Autodesk Fusion 360 part; units mm, degrees
(part 5 of 12)
sketch "草图29" plane through (-71.4999, -0.0001, 0) normal (-1, -0.000001, 0) x (0.000001, -1, 0)
  line L0 (-161.5001, 0) -> (74.9986, 0)
  line L1 (74.9986, 0) -> (74.9986, 250)
  line L2 (74.9986, 250) -> (-161.5001, 250)
  line L3 (-161.5001, 250) -> (-161.5001, 0)
  line L4 (-151.5001, 15) -> (-155.8302, 12.5)
  line L5 (-155.8302, 12.5) -> (-155.8302, 7.5)
  line L6 (-155.8302, 7.5) -> (-151.5001, 5)
  line L7 (-151.5001, 5) -> (-147.17, 7.5)
  line L8 (-147.17, 7.5) -> (-147.17, 12.5)
  line L9 (-147.17, 12.5) -> (-151.5001, 15)
  line L10 (-140.8398, 15) -> (-145.17, 12.5)
  line L11 (-145.17, 12.5) -> (-145.17, 7.5)
  line L12 (-145.17, 7.5) -> (-140.8398, 5)
  line L13 (-140.8398, 5) -> (-136.5097, 7.5)
  line L14 (-136.5097, 7.5) -> (-136.5097, 12.5)
  line L15 (-136.5097, 12.5) -> (-140.8398, 15)
  line L16 (-130.1796, 15) -> (-134.5097, 12.5)
  line L17 (-134.5097, 12.5) -> (-134.5097, 7.5)
  line L18 (-134.5097, 7.5) -> (-130.1796, 5)
  line L19 (-130.1796, 5) -> (-125.8494, 7.5)
  line L20 (-125.8494, 7.5) -> (-125.8494, 12.5)
  line L21 (-125.8494, 12.5) -> (-130.1796, 15)
  line L22 (-119.5193, 15) -> (-123.8494, 12.5)
  line L23 (-123.8494, 12.5) -> (-123.8494, 7.5)
  line L24 (-123.8494, 7.5) -> (-119.5193, 5)
  line L25 (-119.5193, 5) -> (-115.1892, 7.5)
  line L26 (-115.1892, 7.5) -> (-115.1892, 12.5)
  line L27 (-115.1892, 12.5) -> (-119.5193, 15)
  line L28 (-108.8591, 15) -> (-113.1892, 12.5)
  line L29 (-113.1892, 12.5) -> (-113.1892, 7.5)
  line L30 (-113.1892, 7.5) -> (-108.8591, 5)
  line L31 (-108.8591, 5) -> (-104.5289, 7.5)
  line L32 (-104.5289, 7.5) -> (-104.5289, 12.5)
  line L33 (-104.5289, 12.5) -> (-108.8591, 15)
  line L34 (-98.1988, 15) -> (-102.5289, 12.5)
  line L35 (-102.5289, 12.5) -> (-102.5289, 7.5)
  line L36 (-102.5289, 7.5) -> (-98.1988, 5)
  line L37 (-98.1988, 5) -> (-93.8687, 7.5)
  line L38 (-93.8687, 7.5) -> (-93.8687, 12.5)
  line L39 (-93.8687, 12.5) -> (-98.1988, 15)
  line L40 (-87.5386, 15) -> (-91.8687, 12.5)
  line L41 (-91.8687, 12.5) -> (-91.8687, 7.5)
  line L42 (-91.8687, 7.5) -> (-87.5386, 5)
  line L43 (-87.5386, 5) -> (-83.2084, 7.5)
  line L44 (-83.2084, 7.5) -> (-83.2084, 12.5)
  line L45 (-83.2084, 12.5) -> (-87.5386, 15)
  line L46 (-76.8783, 15) -> (-81.2084, 12.5)
  line L47 (-81.2084, 12.5) -> (-81.2084, 7.5)
  line L48 (-81.2084, 7.5) -> (-76.8783, 5)
  line L49 (-76.8783, 5) -> (-72.5482, 7.5)
  line L50 (-72.5482, 7.5) -> (-72.5482, 12.5)
  line L51 (-72.5482, 12.5) -> (-76.8783, 15)
  line L52 (-66.218, 15) -> (-70.5482, 12.5)
  line L53 (-70.5482, 12.5) -> (-70.5482, 7.5)
  line L54 (-70.5482, 7.5) -> (-66.218, 5)
  line L55 (-66.218, 5) -> (-61.8879, 7.5)
  line L56 (-61.8879, 7.5) -> (-61.8879, 12.5)
  line L57 (-61.8879, 12.5) -> (-66.218, 15)
  line L58 (-55.5578, 15) -> (-59.8879, 12.5)
  line L59 (-59.8879, 12.5) -> (-59.8879, 7.5)
  line L60 (-59.8879, 7.5) -> (-55.5578, 5)
  line L61 (-55.5578, 5) -> (-51.2277, 7.5)
  line L62 (-51.2277, 7.5) -> (-51.2277, 12.5)
  line L63 (-51.2277, 12.5) -> (-55.5578, 15)
  line L64 (-44.8975, 15) -> (-49.2277, 12.5)
  line L65 (-49.2277, 12.5) -> (-49.2277, 7.5)
  line L66 (-49.2277, 7.5) -> (-44.8975, 5)
  line L67 (-44.8975, 5) -> (-40.5674, 7.5)
  line L68 (-40.5674, 7.5) -> (-40.5674, 12.5)
  line L69 (-40.5674, 12.5) -> (-44.8975, 15)
  line L70 (-34.2373, 15) -> (-38.5674, 12.5)
  line L71 (-38.5674, 12.5) -> (-38.5674, 7.5)
  line L72 (-38.5674, 7.5) -> (-34.2373, 5)
  line L73 (-34.2373, 5) -> (-29.9072, 7.5)
  line L74 (-29.9072, 7.5) -> (-29.9072, 12.5)
  line L75 (-29.9072, 12.5) -> (-34.2373, 15)
  line L76 (-23.577, 15) -> (-27.9072, 12.5)
  line L77 (-27.9072, 12.5) -> (-27.9072, 7.5)
  line L78 (-27.9072, 7.5) -> (-23.577, 5)
  line L79 (-23.577, 5) -> (-19.2469, 7.5)
  line L80 (-19.2469, 7.5) -> (-19.2469, 12.5)
  line L81 (-19.2469, 12.5) -> (-23.577, 15)
  line L82 (-12.9168, 15) -> (-17.2469, 12.5)
  line L83 (-17.2469, 12.5) -> (-17.2469, 7.5)
  line L84 (-17.2469, 7.5) -> (-12.9168, 5)
  line L85 (-12.9168, 5) -> (-8.5866, 7.5)
  line L86 (-8.5866, 7.5) -> (-8.5866, 12.5)
  line L87 (-8.5866, 12.5) -> (-12.9168, 15)
  line L88 (-2.2565, 15) -> (-6.5866, 12.5)
  line L89 (-6.5866, 12.5) -> (-6.5866, 7.5)
  line L90 (-6.5866, 7.5) -> (-2.2565, 5)
  line L91 (-2.2565, 5) -> (2.0736, 7.5)
  line L92 (2.0736, 7.5) -> (2.0736, 12.5)
  line L93 (2.0736, 12.5) -> (-2.2565, 15)
  line L94 (8.4037, 15) -> (4.0736, 12.5)
  line L95 (4.0736, 12.5) -> (4.0736, 7.5)
  line L96 (4.0736, 7.5) -> (8.4037, 5)
  line L97 (8.4037, 5) -> (12.7339, 7.5)
  line L98 (12.7339, 7.5) -> (12.7339, 12.5)
  line L99 (12.7339, 12.5) -> (8.4037, 15)
  line L100 (19.064, 15) -> (14.7339, 12.5)
  line L101 (14.7339, 12.5) -> (14.7339, 7.5)
  line L102 (14.7339, 7.5) -> (19.064, 5)
  line L103 (19.064, 5) -> (23.3941, 7.5)
  line L104 (23.3941, 7.5) -> (23.3941, 12.5)
  line L105 (23.3941, 12.5) -> (19.064, 15)
  line L106 (29.7242, 15) -> (25.3941, 12.5)
  line L107 (25.3941, 12.5) -> (25.3941, 7.5)
  line L108 (25.3941, 7.5) -> (29.7242, 5)
  line L109 (29.7242, 5) -> (34.0544, 7.5)
  line L110 (34.0544, 7.5) -> (34.0544, 12.5)
  line L111 (34.0544, 12.5) -> (29.7242, 15)
  line L112 (40.3845, 15) -> (36.0544, 12.5)
  line L113 (36.0544, 12.5) -> (36.0544, 7.5)
  line L114 (36.0544, 7.5) -> (40.3845, 5)
  line L115 (40.3845, 5) -> (44.7146, 7.5)
  line L116 (44.7146, 7.5) -> (44.7146, 12.5)
  line L117 (44.7146, 12.5) -> (40.3845, 15)
  line L118 (51.0447, 15) -> (46.7146, 12.5)
  line L119 (46.7146, 12.5) -> (46.7146, 7.5)
  line L120 (46.7146, 7.5) -> (51.0447, 5)
  line L121 (51.0447, 5) -> (55.3749, 7.5)
  line L122 (55.3749, 7.5) -> (55.3749, 12.5)
  line L123 (55.3749, 12.5) -> (51.0447, 15)
  line L124 (61.705, 15) -> (57.3749, 12.5)
  line L125 (57.3749, 12.5) -> (57.3749, 7.5)
  line L126 (57.3749, 7.5) -> (61.705, 5)
  line L127 (61.705, 5) -> (66.0351, 7.5)
  line L128 (66.0351, 7.5) -> (66.0351, 12.5)
  line L129 (66.0351, 12.5) -> (61.705, 15)
  line L130 (-146.17, 24.2321) -> (-150.5001, 21.7321)
  line L131 (-150.5001, 21.7321) -> (-150.5001, 16.7321)
  line L132 (-150.5001, 16.7321) -> (-146.17, 14.2321)
  line L133 (-146.17, 14.2321) -> (-141.8398, 16.7321)
  line L134 (-141.8398, 16.7321) -> (-141.8398, 21.7321)
  line L135 (-141.8398, 21.7321) -> (-146.17, 24.2321)
  line L136 (-135.5097, 24.2321) -> (-139.8398, 21.7321)
  line L137 (-139.8398, 21.7321) -> (-139.8398, 16.7321)
  line L138 (-139.8398, 16.7321) -> (-135.5097, 14.2321)
  line L139 (-135.5097, 14.2321) -> (-131.1796, 16.7321)
  line L140 (-131.1796, 16.7321) -> (-131.1796, 21.7321)
  line L141 (-131.1796, 21.7321) -> (-135.5097, 24.2321)
  line L142 (-124.8494, 24.2321) -> (-129.1796, 21.7321)
  line L143 (-129.1796, 21.7321) -> (-129.1796, 16.7321)
  line L144 (-129.1796, 16.7321) -> (-124.8494, 14.2321)
  line L145 (-124.8494, 14.2321) -> (-120.5193, 16.7321)
  line L146 (-120.5193, 16.7321) -> (-120.5193, 21.7321)
  line L147 (-120.5193, 21.7321) -> (-124.8494, 24.2321)
  line L148 (-114.1892, 24.2321) -> (-118.5193, 21.7321)
  line L149 (-118.5193, 21.7321) -> (-118.5193, 16.7321)
  line L150 (-118.5193, 16.7321) -> (-114.1892, 14.2321)
  line L151 (-114.1892, 14.2321) -> (-109.8591, 16.7321)
  line L152 (-109.8591, 16.7321) -> (-109.8591, 21.7321)
  line L153 (-109.8591, 21.7321) -> (-114.1892, 24.2321)
  line L154 (-103.5289, 24.2321) -> (-107.8591, 21.7321)
  line L155 (-107.8591, 21.7321) -> (-107.8591, 16.7321)
  line L156 (-107.8591, 16.7321) -> (-103.5289, 14.2321)
  line L157 (-103.5289, 14.2321) -> (-99.1988, 16.7321)
  line L158 (-99.1988, 16.7321) -> (-99.1988, 21.7321)
  line L159 (-99.1988, 21.7321) -> (-103.5289, 24.2321)
  line L160 (-92.8687, 24.2321) -> (-97.1988, 21.7321)
  line L161 (-97.1988, 21.7321) -> (-97.1988, 16.7321)
  line L162 (-97.1988, 16.7321) -> (-92.8687, 14.2321)
  line L163 (-92.8687, 14.2321) -> (-88.5386, 16.7321)
  line L164 (-88.5386, 16.7321) -> (-88.5386, 21.7321)
  line L165 (-88.5386, 21.7321) -> (-92.8687, 24.2321)
  line L166 (-82.2084, 24.2321) -> (-86.5386, 21.7321)
  line L167 (-86.5386, 21.7321) -> (-86.5386, 16.7321)
  line L168 (-86.5386, 16.7321) -> (-82.2084, 14.2321)
  line L169 (-82.2084, 14.2321) -> (-77.8783, 16.7321)
  line L170 (-77.8783, 16.7321) -> (-77.8783, 21.7321)
  line L171 (-77.8783, 21.7321) -> (-82.2084, 24.2321)
  line L172 (-71.5482, 24.2321) -> (-75.8783, 21.7321)
  line L173 (-75.8783, 21.7321) -> (-75.8783, 16.7321)
  line L174 (-75.8783, 16.7321) -> (-71.5482, 14.2321)
  line L175 (-71.5482, 14.2321) -> (-67.218, 16.7321)
  line L176 (-67.218, 16.7321) -> (-67.218, 21.7321)
  line L177 (-67.218, 21.7321) -> (-71.5482, 24.2321)
  line L178 (-60.8879, 24.2321) -> (-65.218, 21.7321)
  line L179 (-65.218, 21.7321) -> (-65.218, 16.7321)
  line L180 (-65.218, 16.7321) -> (-60.8879, 14.2321)
  line L181 (-60.8879, 14.2321) -> (-56.5578, 16.7321)
  line L182 (-56.5578, 16.7321) -> (-56.5578, 21.7321)
  line L183 (-56.5578, 21.7321) -> (-60.8879, 24.2321)
  line L184 (-50.2277, 24.2321) -> (-54.5578, 21.7321)
  line L185 (-54.5578, 21.7321) -> (-54.5578, 16.7321)
  line L186 (-54.5578, 16.7321) -> (-50.2277, 14.2321)
  line L187 (-50.2277, 14.2321) -> (-45.8975, 16.7321)
  line L188 (-45.8975, 16.7321) -> (-45.8975, 21.7321)
  line L189 (-45.8975, 21.7321) -> (-50.2277, 24.2321)
  line L190 (-39.5674, 24.2321) -> (-43.8975, 21.7321)
  line L191 (-43.8975, 21.7321) -> (-43.8975, 16.7321)
  line L192 (-43.8975, 16.7321) -> (-39.5674, 14.2321)
  line L193 (-39.5674, 14.2321) -> (-35.2373, 16.7321)
  line L194 (-35.2373, 16.7321) -> (-35.2373, 21.7321)
  line L195 (-35.2373, 21.7321) -> (-39.5674, 24.2321)
  line L196 (-28.9072, 24.2321) -> (-33.2373, 21.7321)
  line L197 (-33.2373, 21.7321) -> (-33.2373, 16.7321)
  line L198 (-33.2373, 16.7321) -> (-28.9072, 14.2321)
  line L199 (-28.9072, 14.2321) -> (-24.577, 16.7321)
  line L200 (-24.577, 16.7321) -> (-24.577, 21.7321)
  line L201 (-24.577, 21.7321) -> (-28.9072, 24.2321)
  line L202 (-18.2469, 24.2321) -> (-22.577, 21.7321)
  line L203 (-22.577, 21.7321) -> (-22.577, 16.7321)
  line L204 (-22.577, 16.7321) -> (-18.2469, 14.2321)
  line L205 (-18.2469, 14.2321) -> (-13.9168, 16.7321)
  line L206 (-13.9168, 16.7321) -> (-13.9168, 21.7321)
  line L207 (-13.9168, 21.7321) -> (-18.2469, 24.2321)
  line L208 (-7.5866, 24.2321) -> (-11.9168, 21.7321)
  line L209 (-11.9168, 21.7321) -> (-11.9168, 16.7321)
  line L210 (-11.9168, 16.7321) -> (-7.5866, 14.2321)
  line L211 (-7.5866, 14.2321) -> (-3.2565, 16.7321)
  line L212 (-3.2565, 16.7321) -> (-3.2565, 21.7321)
  line L213 (-3.2565, 21.7321) -> (-7.5866, 24.2321)
  line L214 (3.0736, 24.2321) -> (-1.2565, 21.7321)
  line L215 (-1.2565, 21.7321) -> (-1.2565, 16.7321)
  line L216 (-1.2565, 16.7321) -> (3.0736, 14.2321)
  line L217 (3.0736, 14.2321) -> (7.4037, 16.7321)
  line L218 (7.4037, 16.7321) -> (7.4037, 21.7321)
  line L219 (7.4037, 21.7321) -> (3.0736, 24.2321)
  line L220 (13.7339, 24.2321) -> (9.4037, 21.7321)
  line L221 (9.4037, 21.7321) -> (9.4037, 16.7321)
  line L222 (9.4037, 16.7321) -> (13.7339, 14.2321)
  line L223 (13.7339, 14.2321) -> (18.064, 16.7321)
  line L224 (18.064, 16.7321) -> (18.064, 21.7321)
  line L225 (18.064, 21.7321) -> (13.7339, 24.2321)
  line L226 (24.3941, 24.2321) -> (20.064, 21.7321)
  line L227 (20.064, 21.7321) -> (20.064, 16.7321)
  line L228 (20.064, 16.7321) -> (24.3941, 14.2321)
  line L229 (24.3941, 14.2321) -> (28.7242, 16.7321)
  line L230 (28.7242, 16.7321) -> (28.7242, 21.7321)
  line L231 (28.7242, 21.7321) -> (24.3941, 24.2321)
  line L232 (35.0544, 24.2321) -> (30.7242, 21.7321)
  line L233 (30.7242, 21.7321) -> (30.7242, 16.7321)
  line L234 (30.7242, 16.7321) -> (35.0544, 14.2321)
  line L235 (35.0544, 14.2321) -> (39.3845, 16.7321)
  line L236 (39.3845, 16.7321) -> (39.3845, 21.7321)
  line L237 (39.3845, 21.7321) -> (35.0544, 24.2321)
  line L238 (45.7146, 24.2321) -> (41.3845, 21.7321)
  line L239 (41.3845, 21.7321) -> (41.3845, 16.7321)
  line L240 (41.3845, 16.7321) -> (45.7146, 14.2321)
  line L241 (45.7146, 14.2321) -> (50.0447, 16.7321)
  line L242 (50.0447, 16.7321) -> (50.0447, 21.7321)
  line L243 (50.0447, 21.7321) -> (45.7146, 24.2321)
  line L244 (56.3749, 24.2321) -> (52.0447, 21.7321)
  line L245 (52.0447, 21.7321) -> (52.0447, 16.7321)
  line L246 (52.0447, 16.7321) -> (56.3749, 14.2321)
  line L247 (56.3749, 14.2321) -> (60.705, 16.7321)
  line L248 (60.705, 16.7321) -> (60.705, 21.7321)
  line L249 (60.705, 21.7321) -> (56.3749, 24.2321)
  line L250 (-151.5001, 33.4641) -> (-155.8302, 30.9641)
  line L251 (-155.8302, 30.9641) -> (-155.8302, 25.9641)
  line L252 (-155.8302, 25.9641) -> (-151.5001, 23.4641)
  line L253 (-151.5001, 23.4641) -> (-147.17, 25.9641)
  line L254 (-147.17, 25.9641) -> (-147.17, 30.9641)
  line L255 (-147.17, 30.9641) -> (-151.5001, 33.4641)
  line L256 (-140.8398, 33.4641) -> (-145.17, 30.9641)
  line L257 (-145.17, 30.9641) -> (-145.17, 25.9641)
  line L258 (-145.17, 25.9641) -> (-140.8398, 23.4641)
  line L259 (-140.8398, 23.4641) -> (-136.5097, 25.9641)
  line L260 (-136.5097, 25.9641) -> (-136.5097, 30.9641)
  line L261 (-136.5097, 30.9641) -> (-140.8398, 33.4641)
  line L262 (-130.1796, 33.4641) -> (-134.5097, 30.9641)
  line L263 (-134.5097, 30.9641) -> (-134.5097, 25.9641)
  line L264 (-134.5097, 25.9641) -> (-130.1796, 23.4641)
  line L265 (-130.1796, 23.4641) -> (-125.8494, 25.9641)
  line L266 (-125.8494, 25.9641) -> (-125.8494, 30.9641)
  line L267 (-125.8494, 30.9641) -> (-130.1796, 33.4641)
  line L268 (-119.5193, 33.4641) -> (-123.8494, 30.9641)
  line L269 (-123.8494, 30.9641) -> (-123.8494, 25.9641)
  line L270 (-123.8494, 25.9641) -> (-119.5193, 23.4641)
  line L271 (-119.5193, 23.4641) -> (-115.1892, 25.9641)
  line L272 (-115.1892, 25.9641) -> (-115.1892, 30.9641)
  line L273 (-115.1892, 30.9641) -> (-119.5193, 33.4641)
  line L274 (-108.8591, 33.4641) -> (-113.1892, 30.9641)
  line L275 (-113.1892, 30.9641) -> (-113.1892, 25.9641)
  line L276 (-113.1892, 25.9641) -> (-108.8591, 23.4641)
  line L277 (-108.8591, 23.4641) -> (-104.5289, 25.9641)
  line L278 (-104.5289, 25.9641) -> (-104.5289, 30.9641)
  line L279 (-104.5289, 30.9641) -> (-108.8591, 33.4641)
  line L280 (-98.1988, 33.4641) -> (-102.5289, 30.9641)
  line L281 (-102.5289, 30.9641) -> (-102.5289, 25.9641)
  line L282 (-102.5289, 25.9641) -> (-98.1988, 23.4641)
  line L283 (-98.1988, 23.4641) -> (-93.8687, 25.9641)
  line L284 (-93.8687, 25.9641) -> (-93.8687, 30.9641)
  line L285 (-93.8687, 30.9641) -> (-98.1988, 33.4641)
  line L286 (-87.5386, 33.4641) -> (-91.8687, 30.9641)
  line L287 (-91.8687, 30.9641) -> (-91.8687, 25.9641)
  line L288 (-91.8687, 25.9641) -> (-87.5386, 23.4641)
  line L289 (-87.5386, 23.4641) -> (-83.2084, 25.9641)
  line L290 (-83.2084, 25.9641) -> (-83.2084, 30.9641)
  line L291 (-83.2084, 30.9641) -> (-87.5386, 33.4641)
  line L292 (-76.8783, 33.4641) -> (-81.2084, 30.9641)
  line L293 (-81.2084, 30.9641) -> (-81.2084, 25.9641)
  line L294 (-81.2084, 25.9641) -> (-76.8783, 23.4641)
  line L295 (-76.8783, 23.4641) -> (-72.5482, 25.9641)
  line L296 (-72.5482, 25.9641) -> (-72.5482, 30.9641)
  line L297 (-72.5482, 30.9641) -> (-76.8783, 33.4641)
  line L298 (-66.218, 33.4641) -> (-70.5482, 30.9641)
  line L299 (-70.5482, 30.9641) -> (-70.5482, 25.9641)
  line L300 (-70.5482, 25.9641) -> (-66.218, 23.4641)
  line L301 (-66.218, 23.4641) -> (-61.8879, 25.9641)
  line L302 (-61.8879, 25.9641) -> (-61.8879, 30.9641)
  line L303 (-61.8879, 30.9641) -> (-66.218, 33.4641)
  line L304 (-55.5578, 33.4641) -> (-59.8879, 30.9641)
  line L305 (-59.8879, 30.9641) -> (-59.8879, 25.9641)
  line L306 (-59.8879, 25.9641) -> (-55.5578, 23.4641)
  line L307 (-55.5578, 23.4641) -> (-51.2277, 25.9641)
  line L308 (-51.2277, 25.9641) -> (-51.2277, 30.9641)
  line L309 (-51.2277, 30.9641) -> (-55.5578, 33.4641)
  line L310 (-44.8975, 33.4641) -> (-49.2277, 30.9641)
  line L311 (-49.2277, 30.9641) -> (-49.2277, 25.9641)
  line L312 (-49.2277, 25.9641) -> (-44.8975, 23.4641)
  line L313 (-44.8975, 23.4641) -> (-40.5674, 25.9641)
  line L314 (-40.5674, 25.9641) -> (-40.5674, 30.9641)
  line L315 (-40.5674, 30.9641) -> (-44.8975, 33.4641)
  line L316 (-34.2373, 33.4641) -> (-38.5674, 30.9641)
  line L317 (-38.5674, 30.9641) -> (-38.5674, 25.9641)
  line L318 (-38.5674, 25.9641) -> (-34.2373, 23.4641)
  line L319 (-34.2373, 23.4641) -> (-29.9072, 25.9641)
  line L320 (-29.9072, 25.9641) -> (-29.9072, 30.9641)
  line L321 (-29.9072, 30.9641) -> (-34.2373, 33.4641)
  line L322 (-23.577, 33.4641) -> (-27.9072, 30.9641)
  line L323 (-27.9072, 30.9641) -> (-27.9072, 25.9641)
  line L324 (-27.9072, 25.9641) -> (-23.577, 23.4641)
  line L325 (-23.577, 23.4641) -> (-19.2469, 25.9641)
  line L326 (-19.2469, 25.9641) -> (-19.2469, 30.9641)
  line L327 (-19.2469, 30.9641) -> (-23.577, 33.4641)
  line L328 (-12.9168, 33.4641) -> (-17.2469, 30.9641)
  line L329 (-17.2469, 30.9641) -> (-17.2469, 25.9641)
  line L330 (-17.2469, 25.9641) -> (-12.9168, 23.4641)
  line L331 (-12.9168, 23.4641) -> (-8.5866, 25.9641)
  line L332 (-8.5866, 25.9641) -> (-8.5866, 30.9641)
  line L333 (-8.5866, 30.9641) -> (-12.9168, 33.4641)
  line L334 (-2.2565, 33.4641) -> (-6.5866, 30.9641)
  line L335 (-6.5866, 30.9641) -> (-6.5866, 25.9641)
  line L336 (-6.5866, 25.9641) -> (-2.2565, 23.4641)
  line L337 (-2.2565, 23.4641) -> (2.0736, 25.9641)
  line L338 (2.0736, 25.9641) -> (2.0736, 30.9641)
  line L339 (2.0736, 30.9641) -> (-2.2565, 33.4641)
  line L340 (8.4037, 33.4641) -> (4.0736, 30.9641)
  line L341 (4.0736, 30.9641) -> (4.0736, 25.9641)
  line L342 (4.0736, 25.9641) -> (8.4037, 23.4641)
  line L343 (8.4037, 23.4641) -> (12.7339, 25.9641)
  line L344 (12.7339, 25.9641) -> (12.7339, 30.9641)
  line L345 (12.7339, 30.9641) -> (8.4037, 33.4641)
  line L346 (19.064, 33.4641) -> (14.7339, 30.9641)
  line L347 (14.7339, 30.9641) -> (14.7339, 25.9641)
  line L348 (14.7339, 25.9641) -> (19.064, 23.4641)
  line L349 (19.064, 23.4641) -> (23.3941, 25.9641)
  line L350 (23.3941, 25.9641) -> (23.3941, 30.9641)
  line L351 (23.3941, 30.9641) -> (19.064, 33.4641)
  line L352 (29.7242, 33.4641) -> (25.3941, 30.9641)
  line L353 (25.3941, 30.9641) -> (25.3941, 25.9641)
  line L354 (25.3941, 25.9641) -> (29.7242, 23.4641)
  line L355 (29.7242, 23.4641) -> (34.0544, 25.9641)
  line L356 (34.0544, 25.9641) -> (34.0544, 30.9641)
  line L357 (34.0544, 30.9641) -> (29.7242, 33.4641)
  line L358 (40.3845, 33.4641) -> (36.0544, 30.9641)
  line L359 (36.0544, 30.9641) -> (36.0544, 25.9641)
  line L360 (36.0544, 25.9641) -> (40.3845, 23.4641)
  line L361 (40.3845, 23.4641) -> (44.7146, 25.9641)
  line L362 (44.7146, 25.9641) -> (44.7146, 30.9641)
  line L363 (44.7146, 30.9641) -> (40.3845, 33.4641)
  line L364 (51.0447, 33.4641) -> (46.7146, 30.9641)
  line L365 (46.7146, 30.9641) -> (46.7146, 25.9641)
  line L366 (46.7146, 25.9641) -> (51.0447, 23.4641)
  line L367 (51.0447, 23.4641) -> (55.3749, 25.9641)
  line L368 (55.3749, 25.9641) -> (55.3749, 30.9641)
  line L369 (55.3749, 30.9641) -> (51.0447, 33.4641)
  line L370 (61.705, 33.4641) -> (57.3749, 30.9641)
  line L371 (57.3749, 30.9641) -> (57.3749, 25.9641)
  line L372 (57.3749, 25.9641) -> (61.705, 23.4641)
  line L373 (61.705, 23.4641) -> (66.0351, 25.9641)
  line L374 (66.0351, 25.9641) -> (66.0351, 30.9641)
  line L375 (66.0351, 30.9641) -> (61.705, 33.4641)
  line L376 (-146.17, 42.6962) -> (-150.5001, 40.1962)
  line L377 (-150.5001, 40.1962) -> (-150.5001, 35.1962)
  line L378 (-150.5001, 35.1962) -> (-146.17, 32.6962)
  line L379 (-146.17, 32.6962) -> (-141.8398, 35.1962)
  line L380 (-141.8398, 35.1962) -> (-141.8398, 40.1962)
  line L381 (-141.8398, 40.1962) -> (-146.17, 42.6962)
  line L382 (-135.5097, 42.6962) -> (-139.8398, 40.1962)
  line L383 (-139.8398, 40.1962) -> (-139.8398, 35.1962)
  line L384 (-139.8398, 35.1962) -> (-135.5097, 32.6962)
  line L385 (-135.5097, 32.6962) -> (-131.1796, 35.1962)
  line L386 (-131.1796, 35.1962) -> (-131.1796, 40.1962)
  line L387 (-131.1796, 40.1962) -> (-135.5097, 42.6962)
  line L388 (-124.8494, 42.6962) -> (-129.1796, 40.1962)
  line L389 (-129.1796, 40.1962) -> (-129.1796, 35.1962)
  line L390 (-129.1796, 35.1962) -> (-124.8494, 32.6962)
  line L391 (-124.8494, 32.6962) -> (-120.5193, 35.1962)
  line L392 (-120.5193, 35.1962) -> (-120.5193, 40.1962)
  line L393 (-120.5193, 40.1962) -> (-124.8494, 42.6962)
  line L394 (-114.1892, 42.6962) -> (-118.5193, 40.1962)
  line L395 (-118.5193, 40.1962) -> (-118.5193, 35.1962)
  line L396 (-118.5193, 35.1962) -> (-114.1892, 32.6962)
  line L397 (-114.1892, 32.6962) -> (-109.8591, 35.1962)
  line L398 (-109.8591, 35.1962) -> (-109.8591, 40.1962)
  line L399 (-109.8591, 40.1962) -> (-114.1892, 42.6962)
  line L400 (-103.5289, 42.6962) -> (-107.8591, 40.1962)
  line L401 (-107.8591, 40.1962) -> (-107.8591, 35.1962)
  line L402 (-107.8591, 35.1962) -> (-103.5289, 32.6962)
  line L403 (-103.5289, 32.6962) -> (-99.1988, 35.1962)
  line L404 (-99.1988, 35.1962) -> (-99.1988, 40.1962)
  line L405 (-99.1988, 40.1962) -> (-103.5289, 42.6962)
  line L406 (-92.8687, 42.6962) -> (-97.1988, 40.1962)
  line L407 (-97.1988, 40.1962) -> (-97.1988, 35.1962)
  line L408 (-97.1988, 35.1962) -> (-92.8687, 32.6962)
  line L409 (-92.8687, 32.6962) -> (-88.5386, 35.1962)
  line L410 (-88.5386, 35.1962) -> (-88.5386, 40.1962)
  line L411 (-88.5386, 40.1962) -> (-92.8687, 42.6962)
  line L412 (-82.2084, 42.6962) -> (-86.5386, 40.1962)
  line L413 (-86.5386, 40.1962) -> (-86.5386, 35.1962)
  line L414 (-86.5386, 35.1962) -> (-82.2084, 32.6962)
  line L415 (-82.2084, 32.6962) -> (-77.8783, 35.1962)
  line L416 (-77.8783, 35.1962) -> (-77.8783, 40.1962)
  line L417 (-77.8783, 40.1962) -> (-82.2084, 42.6962)
  line L418 (-71.5482, 42.6962) -> (-75.8783, 40.1962)
  line L419 (-75.8783, 40.1962) -> (-75.8783, 35.1962)
  line L420 (-75.8783, 35.1962) -> (-71.5482, 32.6962)
  line L421 (-71.5482, 32.6962) -> (-67.218, 35.1962)
  line L422 (-67.218, 35.1962) -> (-67.218, 40.1962)
  line L423 (-67.218, 40.1962) -> (-71.5482, 42.6962)
  line L424 (-60.8879, 42.6962) -> (-65.218, 40.1962)
  line L425 (-65.218, 40.1962) -> (-65.218, 35.1962)
  line L426 (-65.218, 35.1962) -> (-60.8879, 32.6962)
  line L427 (-60.8879, 32.6962) -> (-56.5578, 35.1962)
  line L428 (-56.5578, 35.1962) -> (-56.5578, 40.1962)
  line L429 (-56.5578, 40.1962) -> (-60.8879, 42.6962)
  line L430 (-50.2277, 42.6962) -> (-54.5578, 40.1962)
  line L431 (-54.5578, 40.1962) -> (-54.5578, 35.1962)
  line L432 (-54.5578, 35.1962) -> (-50.2277, 32.6962)
  line L433 (-50.2277, 32.6962) -> (-45.8975, 35.1962)
  line L434 (-45.8975, 35.1962) -> (-45.8975, 40.1962)
  line L435 (-45.8975, 40.1962) -> (-50.2277, 42.6962)
  line L436 (-39.5674, 42.6962) -> (-43.8975, 40.1962)
  line L437 (-43.8975, 40.1962) -> (-43.8975, 35.1962)
  line L438 (-43.8975, 35.1962) -> (-39.5674, 32.6962)
  line L439 (-39.5674, 32.6962) -> (-35.2373, 35.1962)
  line L440 (-35.2373, 35.1962) -> (-35.2373, 40.1962)
  line L441 (-35.2373, 40.1962) -> (-39.5674, 42.6962)
  line L442 (-28.9072, 42.6962) -> (-33.2373, 40.1962)
  line L443 (-33.2373, 40.1962) -> (-33.2373, 35.1962)
  line L444 (-33.2373, 35.1962) -> (-28.9072, 32.6962)
  line L445 (-28.9072, 32.6962) -> (-24.577, 35.1962)
  line L446 (-24.577, 35.1962) -> (-24.577, 40.1962)
  line L447 (-24.577, 40.1962) -> (-28.9072, 42.6962)
  line L448 (-18.2469, 42.6962) -> (-22.577, 40.1962)
  line L449 (-22.577, 40.1962) -> (-22.577, 35.1962)
  line L450 (-22.577, 35.1962) -> (-18.2469, 32.6962)
  line L451 (-18.2469, 32.6962) -> (-13.9168, 35.1962)
  line L452 (-13.9168, 35.1962) -> (-13.9168, 40.1962)
  line L453 (-13.9168, 40.1962) -> (-18.2469, 42.6962)
  line L454 (-7.5866, 42.6962) -> (-11.9168, 40.1962)
  line L455 (-11.9168, 40.1962) -> (-11.9168, 35.1962)
  line L456 (-11.9168, 35.1962) -> (-7.5866, 32.6962)
  line L457 (-7.5866, 32.6962) -> (-3.2565, 35.1962)
  line L458 (-3.2565, 35.1962) -> (-3.2565, 40.1962)
  line L459 (-3.2565, 40.1962) -> (-7.5866, 42.6962)
  line L460 (3.0736, 42.6962) -> (-1.2565, 40.1962)
  line L461 (-1.2565, 40.1962) -> (-1.2565, 35.1962)
  line L462 (-1.2565, 35.1962) -> (3.0736, 32.6962)
  line L463 (3.0736, 32.6962) -> (7.4037, 35.1962)
  line L464 (7.4037, 35.1962) -> (7.4037, 40.1962)
  line L465 (7.4037, 40.1962) -> (3.0736, 42.6962)
  line L466 (13.7339, 42.6962) -> (9.4037, 40.1962)
  line L467 (9.4037, 40.1962) -> (9.4037, 35.1962)
  line L468 (9.4037, 35.1962) -> (13.7339, 32.6962)
  line L469 (13.7339, 32.6962) -> (18.064, 35.1962)
  line L470 (18.064, 35.1962) -> (18.064, 40.1962)
  line L471 (18.064, 40.1962) -> (13.7339, 42.6962)
  line L472 (24.3941, 42.6962) -> (20.064, 40.1962)
  line L473 (20.064, 40.1962) -> (20.064, 35.1962)
  line L474 (20.064, 35.1962) -> (24.3941, 32.6962)
  line L475 (24.3941, 32.6962) -> (28.7242, 35.1962)
  line L476 (28.7242, 35.1962) -> (28.7242, 40.1962)
  line L477 (28.7242, 40.1962) -> (24.3941, 42.6962)
  line L478 (35.0544, 42.6962) -> (30.7242, 40.1962)
  line L479 (30.7242, 40.1962) -> (30.7242, 35.1962)
  line L480 (30.7242, 35.1962) -> (35.0544, 32.6962)
  line L481 (35.0544, 32.6962) -> (39.3845, 35.1962)
  line L482 (39.3845, 35.1962) -> (39.3845, 40.1962)
  line L483 (39.3845, 40.1962) -> (35.0544, 42.6962)
  line L484 (45.7146, 42.6962) -> (41.3845, 40.1962)
  line L485 (41.3845, 40.1962) -> (41.3845, 35.1962)
  line L486 (41.3845, 35.1962) -> (45.7146, 32.6962)
  line L487 (45.7146, 32.6962) -> (50.0447, 35.1962)
  line L488 (50.0447, 35.1962) -> (50.0447, 40.1962)
  line L489 (50.0447, 40.1962) -> (45.7146, 42.6962)
  line L490 (56.3749, 42.6962) -> (52.0447, 40.1962)
  line L491 (52.0447, 40.1962) -> (52.0447, 35.1962)
  line L492 (52.0447, 35.1962) -> (56.3749, 32.6962)
  line L493 (56.3749, 32.6962) -> (60.705, 35.1962)
  line L494 (60.705, 35.1962) -> (60.705, 40.1962)
  line L495 (60.705, 40.1962) -> (56.3749, 42.6962)
  line L496 (-151.5001, 51.9282) -> (-155.8302, 49.4282)
  line L497 (-155.8302, 49.4282) -> (-155.8302, 44.4282)
  line L498 (-155.8302, 44.4282) -> (-151.5001, 41.9282)
  line L499 (-151.5001, 41.9282) -> (-147.17, 44.4282)
  line L500 (-147.17, 44.4282) -> (-147.17, 49.4282)
  line L501 (-147.17, 49.4282) -> (-151.5001, 51.9282)
  line L502 (-140.8398, 51.9282) -> (-145.17, 49.4282)
  line L503 (-145.17, 49.4282) -> (-145.17, 44.4282)
  line L504 (-145.17, 44.4282) -> (-140.8398, 41.9282)
  line L505 (-140.8398, 41.9282) -> (-136.5097, 44.4282)
  line L506 (-136.5097, 44.4282) -> (-136.5097, 49.4282)
  line L507 (-136.5097, 49.4282) -> (-140.8398, 51.9282)
  line L508 (-130.1796, 51.9282) -> (-134.5097, 49.4282)
  line L509 (-134.5097, 49.4282) -> (-134.5097, 44.4282)
  line L510 (-134.5097, 44.4282) -> (-130.1796, 41.9282)
  line L511 (-130.1796, 41.9282) -> (-125.8494, 44.4282)
  line L512 (-125.8494, 44.4282) -> (-125.8494, 49.4282)
  line L513 (-125.8494, 49.4282) -> (-130.1796, 51.9282)
  line L514 (-119.5193, 51.9282) -> (-123.8494, 49.4282)
  line L515 (-123.8494, 49.4282) -> (-123.8494, 44.4282)
  line L516 (-123.8494, 44.4282) -> (-119.5193, 41.9282)
  line L517 (-119.5193, 41.9282) -> (-115.1892, 44.4282)
  line L518 (-115.1892, 44.4282) -> (-115.1892, 49.4282)
  line L519 (-115.1892, 49.4282) -> (-119.5193, 51.9282)
  line L520 (-108.8591, 51.9282) -> (-113.1892, 49.4282)
  line L521 (-113.1892, 49.4282) -> (-113.1892, 44.4282)
  line L522 (-113.1892, 44.4282) -> (-108.8591, 41.9282)
  line L523 (-108.8591, 41.9282) -> (-104.5289, 44.4282)
  line L524 (-104.5289, 44.4282) -> (-104.5289, 49.4282)
  line L525 (-104.5289, 49.4282) -> (-108.8591, 51.9282)
  line L526 (-98.1988, 51.9282) -> (-102.5289, 49.4282)
  line L527 (-102.5289, 49.4282) -> (-102.5289, 44.4282)
  line L528 (-102.5289, 44.4282) -> (-98.1988, 41.9282)
  line L529 (-98.1988, 41.9282) -> (-93.8687, 44.4282)
  line L530 (-93.8687, 44.4282) -> (-93.8687, 49.4282)
  line L531 (-93.8687, 49.4282) -> (-98.1988, 51.9282)
  line L532 (-87.5386, 51.9282) -> (-91.8687, 49.4282)
  line L533 (-91.8687, 49.4282) -> (-91.8687, 44.4282)
  line L534 (-91.8687, 44.4282) -> (-87.5386, 41.9282)
  line L535 (-87.5386, 41.9282) -> (-83.2084, 44.4282)
  line L536 (-83.2084, 44.4282) -> (-83.2084, 49.4282)
  line L537 (-83.2084, 49.4282) -> (-87.5386, 51.9282)
  line L538 (-76.8783, 51.9282) -> (-81.2084, 49.4282)
  line L539 (-81.2084, 49.4282) -> (-81.2084, 44.4282)
  line L540 (-81.2084, 44.4282) -> (-76.8783, 41.9282)
  line L541 (-76.8783, 41.9282) -> (-72.5482, 44.4282)
  line L542 (-72.5482, 44.4282) -> (-72.5482, 49.4282)
  line L543 (-72.5482, 49.4282) -> (-76.8783, 51.9282)
  line L544 (-66.218, 51.9282) -> (-70.5482, 49.4282)
  line L545 (-70.5482, 49.4282) -> (-70.5482, 44.4282)
  line L546 (-70.5482, 44.4282) -> (-66.218, 41.9282)
  line L547 (-66.218, 41.9282) -> (-61.8879, 44.4282)
  line L548 (-61.8879, 44.4282) -> (-61.8879, 49.4282)
  line L549 (-61.8879, 49.4282) -> (-66.218, 51.9282)
  line L550 (-55.5578, 51.9282) -> (-59.8879, 49.4282)
  line L551 (-59.8879, 49.4282) -> (-59.8879, 44.4282)
  line L552 (-59.8879, 44.4282) -> (-55.5578, 41.9282)
  line L553 (-55.5578, 41.9282) -> (-51.2277, 44.4282)
  line L554 (-51.2277, 44.4282) -> (-51.2277, 49.4282)
  line L555 (-51.2277, 49.4282) -> (-55.5578, 51.9282)
  line L556 (-44.8975, 51.9282) -> (-49.2277, 49.4282)
  line L557 (-49.2277, 49.4282) -> (-49.2277, 44.4282)
  line L558 (-49.2277, 44.4282) -> (-44.8975, 41.9282)
  line L559 (-44.8975, 41.9282) -> (-40.5674, 44.4282)
  line L560 (-40.5674, 44.4282) -> (-40.5674, 49.4282)
  line L561 (-40.5674, 49.4282) -> (-44.8975, 51.9282)
  line L562 (-34.2373, 51.9282) -> (-38.5674, 49.4282)
  line L563 (-38.5674, 49.4282) -> (-38.5674, 44.4282)
  line L564 (-38.5674, 44.4282) -> (-34.2373, 41.9282)
  line L565 (-34.2373, 41.9282) -> (-29.9072, 44.4282)
  line L566 (-29.9072, 44.4282) -> (-29.9072, 49.4282)
  line L567 (-29.9072, 49.4282) -> (-34.2373, 51.9282)
  line L568 (-23.577, 51.9282) -> (-27.9072, 49.4282)
  line L569 (-27.9072, 49.4282) -> (-27.9072, 44.4282)
  line L570 (-27.9072, 44.4282) -> (-23.577, 41.9282)
  line L571 (-23.577, 41.9282) -> (-19.2469, 44.4282)
  line L572 (-19.2469, 44.4282) -> (-19.2469, 49.4282)
  line L573 (-19.2469, 49.4282) -> (-23.577, 51.9282)
  line L574 (-12.9168, 51.9282) -> (-17.2469, 49.4282)
  line L575 (-17.2469, 49.4282) -> (-17.2469, 44.4282)
  line L576 (-17.2469, 44.4282) -> (-12.9168, 41.9282)
  line L577 (-12.9168, 41.9282) -> (-8.5866, 44.4282)
  line L578 (-8.5866, 44.4282) -> (-8.5866, 49.4282)
  line L579 (-8.5866, 49.4282) -> (-12.9168, 51.9282)
  line L580 (-2.2565, 51.9282) -> (-6.5866, 49.4282)
  line L581 (-6.5866, 49.4282) -> (-6.5866, 44.4282)
  line L582 (-6.5866, 44.4282) -> (-2.2565, 41.9282)
  line L583 (-2.2565, 41.9282) -> (2.0736, 44.4282)
  line L584 (2.0736, 44.4282) -> (2.0736, 49.4282)
  line L585 (2.0736, 49.4282) -> (-2.2565, 51.9282)
  line L586 (8.4037, 51.9282) -> (4.0736, 49.4282)
  line L587 (4.0736, 49.4282) -> (4.0736, 44.4282)
  line L588 (4.0736, 44.4282) -> (8.4037, 41.9282)
  line L589 (8.4037, 41.9282) -> (12.7339, 44.4282)
  line L590 (12.7339, 44.4282) -> (12.7339, 49.4282)
  line L591 (12.7339, 49.4282) -> (8.4037, 51.9282)
  line L592 (19.064, 51.9282) -> (14.7339, 49.4282)
  line L593 (14.7339, 49.4282) -> (14.7339, 44.4282)
  line L594 (14.7339, 44.4282) -> (19.064, 41.9282)
  line L595 (19.064, 41.9282) -> (23.3941, 44.4282)
  line L596 (23.3941, 44.4282) -> (23.3941, 49.4282)
  line L597 (23.3941, 49.4282) -> (19.064, 51.9282)
  line L598 (29.7242, 51.9282) -> (25.3941, 49.4282)
  line L599 (25.3941, 49.4282) -> (25.3941, 44.4282)
  line L600 (25.3941, 44.4282) -> (29.7242, 41.9282)
  line L601 (29.7242, 41.9282) -> (34.0544, 44.4282)
  line L602 (34.0544, 44.4282) -> (34.0544, 49.4282)
  line L603 (34.0544, 49.4282) -> (29.7242, 51.9282)
  line L604 (40.3845, 51.9282) -> (36.0544, 49.4282)
  line L605 (36.0544, 49.4282) -> (36.0544, 44.4282)
  line L606 (36.0544, 44.4282) -> (40.3845, 41.9282)
  line L607 (40.3845, 41.9282) -> (44.7146, 44.4282)
  line L608 (44.7146, 44.4282) -> (44.7146, 49.4282)
  line L609 (44.7146, 49.4282) -> (40.3845, 51.9282)
  line L610 (51.0447, 51.9282) -> (46.7146, 49.4282)
  line L611 (46.7146, 49.4282) -> (46.7146, 44.4282)
  line L612 (46.7146, 44.4282) -> (51.0447, 41.9282)
  line L613 (51.0447, 41.9282) -> (55.3749, 44.4282)
  line L614 (55.3749, 44.4282) -> (55.3749, 49.4282)
  line L615 (55.3749, 49.4282) -> (51.0447, 51.9282)
  line L616 (61.705, 51.9282) -> (57.3749, 49.4282)
  line L617 (57.3749, 49.4282) -> (57.3749, 44.4282)
  line L618 (57.3749, 44.4282) -> (61.705, 41.9282)
  line L619 (61.705, 41.9282) -> (66.0351, 44.4282)
  line L620 (66.0351, 44.4282) -> (66.0351, 49.4282)
  line L621 (66.0351, 49.4282) -> (61.705, 51.9282)
  line L622 (-146.17, 61.1603) -> (-150.5001, 58.6603)
  line L623 (-150.5001, 58.6603) -> (-150.5001, 53.6603)
  line L624 (-150.5001, 53.6603) -> (-146.17, 51.1603)
  line L625 (-146.17, 51.1603) -> (-141.8398, 53.6603)
  line L626 (-141.8398, 53.6603) -> (-141.8398, 58.6603)
  line L627 (-141.8398, 58.6603) -> (-146.17, 61.1603)
  line L628 (-135.5097, 61.1603) -> (-139.8398, 58.6603)
  line L629 (-139.8398, 58.6603) -> (-139.8398, 53.6603)
  line L630 (-139.8398, 53.6603) -> (-135.5097, 51.1603)
  line L631 (-135.5097, 51.1603) -> (-131.1796, 53.6603)
  line L632 (-131.1796, 53.6603) -> (-131.1796, 58.6603)
  line L633 (-131.1796, 58.6603) -> (-135.5097, 61.1603)
  line L634 (-124.8494, 61.1603) -> (-129.1796, 58.6603)
  line L635 (-129.1796, 58.6603) -> (-129.1796, 53.6603)
  line L636 (-129.1796, 53.6603) -> (-124.8494, 51.1603)
  line L637 (-124.8494, 51.1603) -> (-120.5193, 53.6603)
  line L638 (-120.5193, 53.6603) -> (-120.5193, 58.6603)
  line L639 (-120.5193, 58.6603) -> (-124.8494, 61.1603)
  line L640 (-114.1892, 61.1603) -> (-118.5193, 58.6603)
  line L641 (-118.5193, 58.6603) -> (-118.5193, 53.6603)
  line L642 (-118.5193, 53.6603) -> (-114.1892, 51.1603)
  line L643 (-114.1892, 51.1603) -> (-109.8591, 53.6603)
  line L644 (-109.8591, 53.6603) -> (-109.8591, 58.6603)
  line L645 (-109.8591, 58.6603) -> (-114.1892, 61.1603)
  line L646 (-103.5289, 61.1603) -> (-107.8591, 58.6603)
  line L647 (-107.8591, 58.6603) -> (-107.8591, 53.6603)
  line L648 (-107.8591, 53.6603) -> (-103.5289, 51.1603)
  line L649 (-103.5289, 51.1603) -> (-99.1988, 53.6603)
  line L650 (-99.1988, 53.6603) -> (-99.1988, 58.6603)
  line L651 (-99.1988, 58.6603) -> (-103.5289, 61.1603)
  line L652 (-92.8687, 61.1603) -> (-97.1988, 58.6603)
  line L653 (-97.1988, 58.6603) -> (-97.1988, 53.6603)
  line L654 (-97.1988, 53.6603) -> (-92.8687, 51.1603)
  line L655 (-92.8687, 51.1603) -> (-88.5386, 53.6603)
  line L656 (-88.5386, 53.6603) -> (-88.5386, 58.6603)
  line L657 (-88.5386, 58.6603) -> (-92.8687, 61.1603)
  line L658 (-82.2084, 61.1603) -> (-86.5386, 58.6603)
  line L659 (-86.5386, 58.6603) -> (-86.5386, 53.6603)
  line L660 (-86.5386, 53.6603) -> (-82.2084, 51.1603)
  line L661 (-82.2084, 51.1603) -> (-77.8783, 53.6603)
  line L662 (-77.8783, 53.6603) -> (-77.8783, 58.6603)
  line L663 (-77.8783, 58.6603) -> (-82.2084, 61.1603)
  line L664 (-71.5482, 61.1603) -> (-75.8783, 58.6603)
  line L665 (-75.8783, 58.6603) -> (-75.8783, 53.6603)
  line L666 (-75.8783, 53.6603) -> (-71.5482, 51.1603)
  line L667 (-71.5482, 51.1603) -> (-67.218, 53.6603)
  line L668 (-67.218, 53.6603) -> (-67.218, 58.6603)
  line L669 (-67.218, 58.6603) -> (-71.5482, 61.1603)
  line L670 (-60.8879, 61.1603) -> (-65.218, 58.6603)
  line L671 (-65.218, 58.6603) -> (-65.218, 53.6603)
  line L672 (-65.218, 53.6603) -> (-60.8879, 51.1603)
  line L673 (-60.8879, 51.1603) -> (-56.5578, 53.6603)
  line L674 (-56.5578, 53.6603) -> (-56.5578, 58.6603)
  line L675 (-56.5578, 58.6603) -> (-60.8879, 61.1603)
  line L676 (-50.2277, 61.1603) -> (-54.5578, 58.6603)
  line L677 (-54.5578, 58.6603) -> (-54.5578, 53.6603)
  line L678 (-54.5578, 53.6603) -> (-50.2277, 51.1603)
  line L679 (-50.2277, 51.1603) -> (-45.8975, 53.6603)
  line L680 (-45.8975, 53.6603) -> (-45.8975, 58.6603)
  line L681 (-45.8975, 58.6603) -> (-50.2277, 61.1603)
  line L682 (-39.5674, 61.1603) -> (-43.8975, 58.6603)
  line L683 (-43.8975, 58.6603) -> (-43.8975, 53.6603)
  line L684 (-43.8975, 53.6603) -> (-39.5674, 51.1603)
  line L685 (-39.5674, 51.1603) -> (-35.2373, 53.6603)
  line L686 (-35.2373, 53.6603) -> (-35.2373, 58.6603)
  line L687 (-35.2373, 58.6603) -> (-39.5674, 61.1603)
  line L688 (-28.9072, 61.1603) -> (-33.2373, 58.6603)
  line L689 (-33.2373, 58.6603) -> (-33.2373, 53.6603)
  line L690 (-33.2373, 53.6603) -> (-28.9072, 51.1603)
  line L691 (-28.9072, 51.1603) -> (-24.577, 53.6603)
  line L692 (-24.577, 53.6603) -> (-24.577, 58.6603)
  line L693 (-24.577, 58.6603) -> (-28.9072, 61.1603)
  line L694 (-18.2469, 61.1603) -> (-22.577, 58.6603)
  line L695 (-22.577, 58.6603) -> (-22.577, 53.6603)
  line L696 (-22.577, 53.6603) -> (-18.2469, 51.1603)
  line L697 (-18.2469, 51.1603) -> (-13.9168, 53.6603)
  line L698 (-13.9168, 53.6603) -> (-13.9168, 58.6603)
  line L699 (-13.9168, 58.6603) -> (-18.2469, 61.1603)
  line L700 (-7.5866, 61.1603) -> (-11.9168, 58.6603)
  line L701 (-11.9168, 58.6603) -> (-11.9168, 53.6603)
  line L702 (-11.9168, 53.6603) -> (-7.5866, 51.1603)
  line L703 (-7.5866, 51.1603) -> (-3.2565, 53.6603)
  line L704 (-3.2565, 53.6603) -> (-3.2565, 58.6603)
  line L705 (-3.2565, 58.6603) -> (-7.5866, 61.1603)
  line L706 (3.0736, 61.1603) -> (-1.2565, 58.6603)
  line L707 (-1.2565, 58.6603) -> (-1.2565, 53.6603)
  line L708 (-1.2565, 53.6603) -> (3.0736, 51.1603)
  line L709 (3.0736, 51.1603) -> (7.4037, 53.6603)
  line L710 (7.4037, 53.6603) -> (7.4037, 58.6603)
  line L711 (7.4037, 58.6603) -> (3.0736, 61.1603)
  line L712 (13.7339, 61.1603) -> (9.4037, 58.6603)
  line L713 (9.4037, 58.6603) -> (9.4037, 53.6603)
  line L714 (9.4037, 53.6603) -> (13.7339, 51.1603)
  line L715 (13.7339, 51.1603) -> (18.064, 53.6603)
  line L716 (18.064, 53.6603) -> (18.064, 58.6603)
  line L717 (18.064, 58.6603) -> (13.7339, 61.1603)
  line L718 (24.3941, 61.1603) -> (20.064, 58.6603)
  line L719 (20.064, 58.6603) -> (20.064, 53.6603)
  line L720 (20.064, 53.6603) -> (24.3941, 51.1603)
  line L721 (24.3941, 51.1603) -> (28.7242, 53.6603)
  line L722 (28.7242, 53.6603) -> (28.7242, 58.6603)
  line L723 (28.7242, 58.6603) -> (24.3941, 61.1603)
  line L724 (35.0544, 61.1603) -> (30.7242, 58.6603)
  line L725 (30.7242, 58.6603) -> (30.7242, 53.6603)
  line L726 (30.7242, 53.6603) -> (35.0544, 51.1603)
  line L727 (35.0544, 51.1603) -> (39.3845, 53.6603)
  line L728 (39.3845, 53.6603) -> (39.3845, 58.6603)
  line L729 (39.3845, 58.6603) -> (35.0544, 61.1603)
  line L730 (45.7146, 61.1603) -> (41.3845, 58.6603)
  line L731 (41.3845, 58.6603) -> (41.3845, 53.6603)
  line L732 (41.3845, 53.6603) -> (45.7146, 51.1603)
  line L733 (45.7146, 51.1603) -> (50.0447, 53.6603)
  line L734 (50.0447, 53.6603) -> (50.0447, 58.6603)
  line L735 (50.0447, 58.6603) -> (45.7146, 61.1603)
  line L736 (56.3749, 61.1603) -> (52.0447, 58.6603)
  line L737 (52.0447, 58.6603) -> (52.0447, 53.6603)
  line L738 (52.0447, 53.6603) -> (56.3749, 51.1603)
  line L739 (56.3749, 51.1603) -> (60.705, 53.6603)
  line L740 (60.705, 53.6603) -> (60.705, 58.6603)
  line L741 (60.705, 58.6603) -> (56.3749, 61.1603)
  line L742 (-151.5001, 70.3923) -> (-155.8302, 67.8923)
  line L743 (-155.8302, 67.8923) -> (-155.8302, 62.8923)
  line L744 (-155.8302, 62.8923) -> (-151.5001, 60.3923)
  line L745 (-151.5001, 60.3923) -> (-147.17, 62.8923)
  line L746 (-147.17, 62.8923) -> (-147.17, 67.8923)
  line L747 (-147.17, 67.8923) -> (-151.5001, 70.3923)
  line L748 (-140.8398, 70.3923) -> (-145.17, 67.8923)
  line L749 (-145.17, 67.8923) -> (-145.17, 62.8923)
  line L750 (-145.17, 62.8923) -> (-140.8398, 60.3923)
  line L751 (-140.8398, 60.3923) -> (-136.5097, 62.8923)
  line L752 (-136.5097, 62.8923) -> (-136.5097, 67.8923)
  line L753 (-136.5097, 67.8923) -> (-140.8398, 70.3923)
  line L754 (-130.1796, 70.3923) -> (-134.5097, 67.8923)
  line L755 (-134.5097, 67.8923) -> (-134.5097, 62.8923)
  line L756 (-134.5097, 62.8923) -> (-130.1796, 60.3923)
  line L757 (-130.1796, 60.3923) -> (-125.8494, 62.8923)
  line L758 (-125.8494, 62.8923) -> (-125.8494, 67.8923)
  line L759 (-125.8494, 67.8923) -> (-130.1796, 70.3923)
  line L760 (-119.5193, 70.3923) -> (-123.8494, 67.8923)
  line L761 (-123.8494, 67.8923) -> (-123.8494, 62.8923)
  line L762 (-123.8494, 62.8923) -> (-119.5193, 60.3923)
  line L763 (-119.5193, 60.3923) -> (-115.1892, 62.8923)
  line L764 (-115.1892, 62.8923) -> (-115.1892, 67.8923)
  line L765 (-115.1892, 67.8923) -> (-119.5193, 70.3923)
  line L766 (-108.8591, 70.3923) -> (-113.1892, 67.8923)
  line L767 (-113.1892, 67.8923) -> (-113.1892, 62.8923)
  line L768 (-113.1892, 62.8923) -> (-108.8591, 60.3923)
  line L769 (-108.8591, 60.3923) -> (-104.5289, 62.8923)
  line L770 (-104.5289, 62.8923) -> (-104.5289, 67.8923)
  line L771 (-104.5289, 67.8923) -> (-108.8591, 70.3923)
  line L772 (-98.1988, 70.3923) -> (-102.5289, 67.8923)
  line L773 (-102.5289, 67.8923) -> (-102.5289, 62.8923)
  line L774 (-102.5289, 62.8923) -> (-98.1988, 60.3923)
  line L775 (-98.1988, 60.3923) -> (-93.8687, 62.8923)
  line L776 (-93.8687, 62.8923) -> (-93.8687, 67.8923)
  line L777 (-93.8687, 67.8923) -> (-98.1988, 70.3923)
  line L778 (-87.5386, 70.3923) -> (-91.8687, 67.8923)
  line L779 (-91.8687, 67.8923) -> (-91.8687, 62.8923)
  line L780 (-91.8687, 62.8923) -> (-87.5386, 60.3923)
  line L781 (-87.5386, 60.3923) -> (-83.2084, 62.8923)
  line L782 (-83.2084, 62.8923) -> (-83.2084, 67.8923)
  line L783 (-83.2084, 67.8923) -> (-87.5386, 70.3923)
  line L784 (-76.8783, 70.3923) -> (-81.2084, 67.8923)
  line L785 (-81.2084, 67.8923) -> (-81.2084, 62.8923)
  line L786 (-81.2084, 62.8923) -> (-76.8783, 60.3923)
  line L787 (-76.8783, 60.3923) -> (-72.5482, 62.8923)
  line L788 (-72.5482, 62.8923) -> (-72.5482, 67.8923)
  line L789 (-72.5482, 67.8923) -> (-76.8783, 70.3923)
  line L790 (-66.218, 70.3923) -> (-70.5482, 67.8923)
  line L791 (-70.5482, 67.8923) -> (-70.5482, 62.8923)
  line L792 (-70.5482, 62.8923) -> (-66.218, 60.3923)
  line L793 (-66.218, 60.3923) -> (-61.8879, 62.8923)
  line L794 (-61.8879, 62.8923) -> (-61.8879, 67.8923)
  line L795 (-61.8879, 67.8923) -> (-66.218, 70.3923)
  line L796 (-55.5578, 70.3923) -> (-59.8879, 67.8923)
  line L797 (-59.8879, 67.8923) -> (-59.8879, 62.8923)
  line L798 (-59.8879, 62.8923) -> (-55.5578, 60.3923)
  line L799 (-55.5578, 60.3923) -> (-51.2277, 62.8923)
  line L800 (-51.2277, 62.8923) -> (-51.2277, 67.8923)
  line L801 (-51.2277, 67.8923) -> (-55.5578, 70.3923)
  line L802 (-44.8975, 70.3923) -> (-49.2277, 67.8923)
  line L803 (-49.2277, 67.8923) -> (-49.2277, 62.8923)
  line L804 (-49.2277, 62.8923) -> (-44.8975, 60.3923)
  line L805 (-44.8975, 60.3923) -> (-40.5674, 62.8923)
  line L806 (-40.5674, 62.8923) -> (-40.5674, 67.8923)
  line L807 (-40.5674, 67.8923) -> (-44.8975, 70.3923)
  line L808 (-34.2373, 70.3923) -> (-38.5674, 67.8923)
  line L809 (-38.5674, 67.8923) -> (-38.5674, 62.8923)
  line L810 (-38.5674, 62.8923) -> (-34.2373, 60.3923)
  line L811 (-34.2373, 60.3923) -> (-29.9072, 62.8923)
  line L812 (-29.9072, 62.8923) -> (-29.9072, 67.8923)
  line L813 (-29.9072, 67.8923) -> (-34.2373, 70.3923)
  line L814 (-23.577, 70.3923) -> (-27.9072, 67.8923)
  line L815 (-27.9072, 67.8923) -> (-27.9072, 62.8923)
  line L816 (-27.9072, 62.8923) -> (-23.577, 60.3923)
  line L817 (-23.577, 60.3923) -> (-19.2469, 62.8923)
  line L818 (-19.2469, 62.8923) -> (-19.2469, 67.8923)
  line L819 (-19.2469, 67.8923) -> (-23.577, 70.3923)
  line L820 (-12.9168, 70.3923) -> (-17.2469, 67.8923)
  line L821 (-17.2469, 67.8923) -> (-17.2469, 62.8923)
  line L822 (-17.2469, 62.8923) -> (-12.9168, 60.3923)
  line L823 (-12.9168, 60.3923) -> (-8.5866, 62.8923)
  line L824 (-8.5866, 62.8923) -> (-8.5866, 67.8923)
  line L825 (-8.5866, 67.8923) -> (-12.9168, 70.3923)
  line L826 (-2.2565, 70.3923) -> (-6.5866, 67.8923)
  line L827 (-6.5866, 67.8923) -> (-6.5866, 62.8923)
  line L828 (-6.5866, 62.8923) -> (-2.2565, 60.3923)
  line L829 (-2.2565, 60.3923) -> (2.0736, 62.8923)
  line L830 (2.0736, 62.8923) -> (2.0736, 67.8923)
  line L831 (2.0736, 67.8923) -> (-2.2565, 70.3923)
  line L832 (8.4037, 70.3923) -> (4.0736, 67.8923)
  line L833 (4.0736, 67.8923) -> (4.0736, 62.8923)
  line L834 (4.0736, 62.8923) -> (8.4037, 60.3923)
  line L835 (8.4037, 60.3923) -> (12.7339, 62.8923)
  line L836 (12.7339, 62.8923) -> (12.7339, 67.8923)
  line L837 (12.7339, 67.8923) -> (8.4037, 70.3923)
  line L838 (19.064, 70.3923) -> (14.7339, 67.8923)
  line L839 (14.7339, 67.8923) -> (14.7339, 62.8923)
  line L840 (14.7339, 62.8923) -> (19.064, 60.3923)
  line L841 (19.064, 60.3923) -> (23.3941, 62.8923)
  line L842 (23.3941, 62.8923) -> (23.3941, 67.8923)
  line L843 (23.3941, 67.8923) -> (19.064, 70.3923)
  line L844 (29.7242, 70.3923) -> (25.3941, 67.8923)
  line L845 (25.3941, 67.8923) -> (25.3941, 62.8923)
  line L846 (25.3941, 62.8923) -> (29.7242, 60.3923)
  line L847 (29.7242, 60.3923) -> (34.0544, 62.8923)
  line L848 (34.0544, 62.8923) -> (34.0544, 67.8923)
  line L849 (34.0544, 67.8923) -> (29.7242, 70.3923)
  line L850 (40.3845, 70.3923) -> (36.0544, 67.8923)
  line L851 (36.0544, 67.8923) -> (36.0544, 62.8923)
  line L852 (36.0544, 62.8923) -> (40.3845, 60.3923)
  line L853 (40.3845, 60.3923) -> (44.7146, 62.8923)
  line L854 (44.7146, 62.8923) -> (44.7146, 67.8923)
  line L855 (44.7146, 67.8923) -> (40.3845, 70.3923)
  line L856 (51.0447, 70.3923) -> (46.7146, 67.8923)
  line L857 (46.7146, 67.8923) -> (46.7146, 62.8923)
  line L858 (46.7146, 62.8923) -> (51.0447, 60.3923)
  line L859 (51.0447, 60.3923) -> (55.3749, 62.8923)
  line L860 (55.3749, 62.8923) -> (55.3749, 67.8923)
  line L861 (55.3749, 67.8923) -> (51.0447, 70.3923)
  line L862 (61.705, 70.3923) -> (57.3749, 67.8923)
  line L863 (57.3749, 67.8923) -> (57.3749, 62.8923)
  line L864 (57.3749, 62.8923) -> (61.705, 60.3923)
  line L865 (61.705, 60.3923) -> (66.0351, 62.8923)
  line L866 (66.0351, 62.8923) -> (66.0351, 67.8923)
  line L867 (66.0351, 67.8923) -> (61.705, 70.3923)
  line L868 (-146.17, 79.6244) -> (-150.5001, 77.1244)
  line L869 (-150.5001, 77.1244) -> (-150.5001, 72.1244)
  line L870 (-150.5001, 72.1244) -> (-146.17, 69.6244)
  line L871 (-146.17, 69.6244) -> (-141.8398, 72.1244)
  line L872 (-141.8398, 72.1244) -> (-141.8398, 77.1244)
  line L873 (-141.8398, 77.1244) -> (-146.17, 79.6244)
  line L874 (-135.5097, 79.6244) -> (-139.8398, 77.1244)
  line L875 (-139.8398, 77.1244) -> (-139.8398, 72.1244)
  line L876 (-139.8398, 72.1244) -> (-135.5097, 69.6244)
  line L877 (-135.5097, 69.6244) -> (-131.1796, 72.1244)
  line L878 (-131.1796, 72.1244) -> (-131.1796, 77.1244)
  line L879 (-131.1796, 77.1244) -> (-135.5097, 79.6244)
  line L880 (-124.8494, 79.6244) -> (-129.1796, 77.1244)
  line L881 (-129.1796, 77.1244) -> (-129.1796, 72.1244)
  line L882 (-129.1796, 72.1244) -> (-124.8494, 69.6244)
  line L883 (-124.8494, 69.6244) -> (-120.5193, 72.1244)
  line L884 (-120.5193, 72.1244) -> (-120.5193, 77.1244)
  line L885 (-120.5193, 77.1244) -> (-124.8494, 79.6244)
  line L886 (-114.1892, 79.6244) -> (-118.5193, 77.1244)
  line L887 (-118.5193, 77.1244) -> (-118.5193, 72.1244)
  line L888 (-118.5193, 72.1244) -> (-114.1892, 69.6244)
  line L889 (-114.1892, 69.6244) -> (-109.8591, 72.1244)
  line L890 (-109.8591, 72.1244) -> (-109.8591, 77.1244)
  line L891 (-109.8591, 77.1244) -> (-114.1892, 79.6244)
  line L892 (-103.5289, 79.6244) -> (-107.8591, 77.1244)
  line L893 (-107.8591, 77.1244) -> (-107.8591, 72.1244)
  line L894 (-107.8591, 72.1244) -> (-103.5289, 69.6244)
  line L895 (-103.5289, 69.6244) -> (-99.1988, 72.1244)
  line L896 (-99.1988, 72.1244) -> (-99.1988, 77.1244)
  line L897 (-99.1988, 77.1244) -> (-103.5289, 79.6244)
  line L898 (-92.8687, 79.6244) -> (-97.1988, 77.1244)
  line L899 (-97.1988, 77.1244) -> (-97.1988, 72.1244)
  line L900 (-97.1988, 72.1244) -> (-92.8687, 69.6244)
  line L901 (-92.8687, 69.6244) -> (-88.5386, 72.1244)
  line L902 (-88.5386, 72.1244) -> (-88.5386, 77.1244)
  line L903 (-88.5386, 77.1244) -> (-92.8687, 79.6244)
  line L904 (-82.2084, 79.6244) -> (-86.5386, 77.1244)
  line L905 (-86.5386, 77.1244) -> (-86.5386, 72.1244)
  line L906 (-86.5386, 72.1244) -> (-82.2084, 69.6244)
  line L907 (-82.2084, 69.6244) -> (-77.8783, 72.1244)
  line L908 (-77.8783, 72.1244) -> (-77.8783, 77.1244)
  line L909 (-77.8783, 77.1244) -> (-82.2084, 79.6244)
  line L910 (-71.5482, 79.6244) -> (-75.8783, 77.1244)
  line L911 (-75.8783, 77.1244) -> (-75.8783, 72.1244)
  line L912 (-75.8783, 72.1244) -> (-71.5482, 69.6244)
  line L913 (-71.5482, 69.6244) -> (-67.218, 72.1244)
  line L914 (-67.218, 72.1244) -> (-67.218, 77.1244)
  line L915 (-67.218, 77.1244) -> (-71.5482, 79.6244)
  line L916 (-60.8879, 79.6244) -> (-65.218, 77.1244)
  line L917 (-65.218, 77.1244) -> (-65.218, 72.1244)
  line L918 (-65.218, 72.1244) -> (-60.8879, 69.6244)
  line L919 (-60.8879, 69.6244) -> (-56.5578, 72.1244)
  line L920 (-56.5578, 72.1244) -> (-56.5578, 77.1244)
  line L921 (-56.5578, 77.1244) -> (-60.8879, 79.6244)
  line L922 (-50.2277, 79.6244) -> (-54.5578, 77.1244)
  line L923 (-54.5578, 77.1244) -> (-54.5578, 72.1244)
  line L924 (-54.5578, 72.1244) -> (-50.2277, 69.6244)
  line L925 (-50.2277, 69.6244) -> (-45.8975, 72.1244)
  line L926 (-45.8975, 72.1244) -> (-45.8975, 77.1244)
  line L927 (-45.8975, 77.1244) -> (-50.2277, 79.6244)
  line L928 (-39.5674, 79.6244) -> (-43.8975, 77.1244)
  line L929 (-43.8975, 77.1244) -> (-43.8975, 72.1244)
  line L930 (-43.8975, 72.1244) -> (-39.5674, 69.6244)
  line L931 (-39.5674, 69.6244) -> (-35.2373, 72.1244)
  line L932 (-35.2373, 72.1244) -> (-35.2373, 77.1244)
  line L933 (-35.2373, 77.1244) -> (-39.5674, 79.6244)
  line L934 (-28.9072, 79.6244) -> (-33.2373, 77.1244)